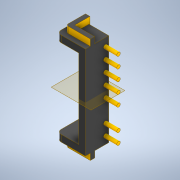
# Autodesk Inventor part: battery_header 7P
Saved by Autodesk Inventor 2022 (Build 260153000, 153)
## iProperties
Created: 2022-07-18
Part Number: battery_header 7P
Material: Типовые
Document SubType Name: Modeling
Designer: akapu
Density: 1 g/cm^3
Appearance: По умолчанию
Author: akapu
Autodesk Inventor part; units mm, degrees
ref_plane "YZ Plane" through (0, 0, 0) normal (1, 0, 0) x (0, 1, 0)
ref_plane "XZ Plane" through (0, 0, 0) normal (0, 1, 0) x (-1, 0, 0)
ref_plane "XY Plane" through (0, 0, 0) normal (0, 0, 1) x (1, 0, 0)
sketch "Эскиз1" plane through (0, 0, 0) normal (0, 1, 0) x (-1, 0, 0)
  line L0 (0, -5) -> (-1, -5)
  line L1 (-1, -5) -> (-3, -5)
  line L2 (-1, -5) -> (-6.5, -5)
  line L3 (-6.5, -5) -> (-6.5, -5)
  line L4 (0, -5) -> (0, -1)
  line L5 (-1, 0) -> (-6.5, 0)
  line L6 (-6.5, 0) -> (-6.5, -5)
  line L7 (-1, -5) -> (-1, -1.1)
  line L8 (-1.5, -0.6) -> (-6.5, -0.6)
  line L9 (-6.5, -0.6) -> (-6.5, -5)
  line L10 (-2, -5) -> (-2, -1.6)
  line L11 (-2, -1.6) -> (-5.5, -1.6)
  line L12 (-5.5, -1.6) -> (-5.5, -5.52)
  line L13 (-5.5, -1.6) -> (-6.5, -1.6)
  arc A0 (0, -1) -> (-1, 0) centre (-1, -1) ccw
  arc A1 (-1, -1.1) -> (-1.5, -0.6) centre (-1.5, -1.1) ccw
  point P0 (0, 0)
  point P1 (0, 0)
  point P2 (-1, -0.6)
  point P3 (-4.25, -5.52)
  dimension "d2" = 1
  dimension "d31" = 5
  dimension "d32" = 4.4
  dimension "d74" = 6.5
  dimension "d75" = 1
  dimension "d76" = 1
  dimension "d77" = 0.5
  constraints: 28 end point, 6 perpendicular, 5 point on line, 4 point on circle, 4 tangent, 3 collinear, 2 centre point, 2 vertical, 1 coincident, 1 horizontal, 2 other
  measures "d2" distance of L0.start L0.end
  measures "d31" distance of L0.start point (0, 0)
  measures "d32" distance of L0.end point (-1, -0.6)
  measures "d74" distance between parallel lines of L4 L6
  measures "d75" distance between parallel lines of L7 L10
  measures "d76" radius of A0
  measures "d77" radius of A1
extrude "Выдавливание1" add sketch "Эскиз1" along normal blind 21
sketch "Эскиз2" plane through (0, 21, 0) normal (0, 1, 0) x (1, 0, 0)
  line L0 (6.5, 5.52) -> (1, 5.52)
  line L1 (1, 5.52) -> (1, 1.62)
  line L2 (1.5, 1.12) -> (6.5, 1.12)
  line L3 (6.5, 1.12) -> (6.5, 5.52)
  line L4 (6.5, 5) -> (0, 5) projected
  line L5 (2, 2.12) -> (2, 4.52)
  line L6 (2, 4.52) -> (5.5, 4.52)
  line L7 (5.5, 4.52) -> (5.5, 2.12)
  line L8 (5.5, 2.12) -> (2, 2.12)
  line L9 (6.5, 5.52) -> (2, 5.52)
  line L10 (2, 5.52) -> (2, 2.12)
  line L11 (2, 2.12) -> (6.5, 2.12)
  line L12 (6.5, 2.12) -> (6.5, 5.52)
  arc A0 (1, 1.62) -> (1.5, 1.12) centre (1.5, 1.62) ccw
  point P0 (0, 0)
  point P1 (1, 1.12)
  point P2 (2, 5)
  point P3 (1, 5)
  point P4 (2, 5.52)
  dimension "d78" = 5.5
  dimension "d79" = 4.4
  dimension "d80" = 0.52
  dimension "d81" = 1
  dimension "d82" = 0.5
  constraints: 24 end point, 6 parallel, 3 perpendicular, 2 horizontal, 2 point on circle, 2 point on line, 2 tangent, 1 centre point, 3 other
  measures "d78" distance of L2.end point (1, 1.12)
  measures "d79" distance of point (1, 1.12) L0.end
  measures "d80" distance between parallel lines of L0 L4
  measures "d81" distance between parallel lines of L1 L5
  measures "d82" radius of A0
extrude "Выдавливание2" add sketch "Эскиз2" along normal blind 1.425 and the other way blind 22.425 contours L10 L4 L1 L0 | L10 L5 L8 L11 L3 L2 A0 L1 L4
sketch "Эскиз6" plane through (0, 0, 0) normal (0, 0, 1) x (1, 0, 0)
  line L0 (0, 0) -> (0, 1.5)
  line L1 (0, 0) -> (0, 21) projected
  line L2 (0, 21) -> (6.5, 21) projected
  line L3 (0, 21) -> (0, 19.5)
  line L4 (0, 19.5) -> (5, 19.5)
  line L5 (5, 19.5) -> (5, 1.5)
  line L6 (5, 1.5) -> (0, 1.5)
  line L7 (0, 1.5) -> (0, 19.5)
  dimension "d33" = 1.5
  dimension "d34" = 1.5
  dimension "d35" = 5
  constraints: 12 end point, 3 perpendicular, 2 point on line, 1 collinear
  measures "d33" distance of L0.start L0.end
  measures "d34" distance of L1.end L3.end
  measures "d35" distance of L3.end L4.end
extrude "Выдавливание5" cut sketch "Эскиз6" against normal blind 5
sketch "Эскиз7" plane through (6.5, 0, 0) normal (1, 0, 0) x (0, 0, -1)
  line L0 (0, 0) -> (0, 21) projected
  line L1 (2.12, 21) -> (5, 21) projected
  line L2 (0, 0) -> (5, 0)
  line L3 (5, 0) -> (5, 21)
  line L4 (5, 21) -> (0, 21)
  line L5 (0, 21) -> (0, 0)
  line L6 (5, 0) -> (5, 21) projected
  line L7 (0, 19.5) -> (0, 1.5) projected
  line L8 (4.52, 10.5) -> (4.52, 19.25)
  line L9 (4.52, 19.25) -> (4.52, 1.75)
  line L10 (5, 10.5) -> (0, 10.5)
  line L11 (4.52, 19.25) -> (4.52, 16.75)
  line L12 (4.52, 16.75) -> (4.52, 14.25)
  line L13 (4.52, 14.25) -> (4.52, 11.75)
  line L14 (4.52, 11.75) -> (4.52, 9.25)
  line L15 (4.52, 9.25) -> (4.52, 6.75)
  line L16 (4.52, 6.75) -> (4.52, 4.25)
  circle A0 centre (4.52, 4.25) radius 0.4
  circle A1 centre (4.52, 1.75) radius 0.4
  circle A2 centre (4.52, 9.25) radius 0.4
  circle A3 centre (4.52, 11.75) radius 0.4
  circle A4 centre (4.52, 14.25) radius 0.4
  circle A5 centre (4.52, 16.75) radius 0.4
  circle A6 centre (4.52, 19.25) radius 0.4
  line L17 (5.52, -1.425) -> (5.52, 22.425) projected
  dimension "d84" = 17.5
  dimension "d85" = 2.5
  dimension "d86" = 2.5
  dimension "d87" = 2.5
  dimension "d88" = 2.5
  dimension "d89" = 2.5
  dimension "d90" = 2.5
  dimension "d91" = 0.8
  dimension "d92" = 0.8
  dimension "d93" = 0.8
  dimension "d94" = 0.8
  dimension "d95" = 0.8
  dimension "d96" = 0.8
  dimension "d97" = 0.8
  dimension "d101" = 1
  constraints: 24 end point, 7 centre point, 7 coincident, 2 midpoint, 2 parallel, 2 point on line, 1 horizontal, 1 perpendicular, 1 vertical, 10 other
  measures "d84" distance of L8.end point (4.52, 1.75)
  measures "d85" distance of L8.end L11.end
  measures "d86" distance of L11.end L12.end
  measures "d87" distance of L12.end L13.end
  measures "d88" distance of L13.end L14.end
  measures "d89" distance of L14.end L15.end
  measures "d90" distance of L15.end L16.end
  measures "d91" diameter of A0
  measures "d92" diameter of A1
  measures "d93" diameter of A2
  measures "d94" diameter of A3
  measures "d95" diameter of A4
  measures "d96" diameter of A5
  measures "d97" diameter of A6
extrude "Выдавливание6" add sketch "Эскиз7" along normal blind 3 contours A1 | A0 L9 | L9 A0 | A2 L9 | L9 A2 | A6 | A5 L8 | L8 A5 | A4 L8 | L8 A4 | A3 L8 | L8 A3
ref_plane "РабПлоскость1" through (0, 10.5, 0) normal (0, 1, 0) x (1, 0, 0)
sketch "Эскиз10" plane through (0, 21, 0) normal (0, 1, 0) x (1, 0, 0)
  line L0 (6.5, 5) -> (2, 5) projected
  line L1 (2, 2.12) -> (2, 5.52) projected
  line L2 (6.5, 5) -> (2, 5)
  line L3 (2, 5) -> (2, 5.3)
  line L4 (2, 5.3) -> (6.5, 5.3)
  line L5 (6.5, 5.3) -> (6.5, 5)
  point P0 (0, 0)
  dimension "d98" = 0.3
  constraints: 8 end point, 2 parallel, 1 horizontal, 1 perpendicular, 1 point on line
  measures "d98" distance of L2.end L3.end
extrude "Выдавливание7" add sketch "Эскиз10" against normal up to surface (21 mm away)
